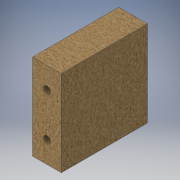
# Autodesk Inventor part: KugelRadStützen
Saved by Autodesk Inventor 2017 SP1 (Build 210196100, 196)
## iProperties
Part Number: KugelRadStützen
Material: Generisch
Document SubType Name: Modeling
Designer: Alex
Density: 1 g/cm^3
Appearance: Vorgabe
Author: Alex
Autodesk Inventor part; units mm, degrees
ref_plane "YZ Plane" through (0, 0, 0) normal (1, 0, 0) x (0, 1, 0)
ref_plane "XZ Plane" through (0, 0, 0) normal (0, 1, 0) x (-1, 0, 0)
ref_plane "XY Plane" through (0, 0, 0) normal (0, 0, 1) x (1, 0, 0)
sketch "Skizze1" plane through (0, 0, 0) normal (0, 1, 0) x (-1, 0, 0)
  line L0 (0, 0) -> (10, 0)
  line L1 (10, 0) -> (10, -30)
  line L2 (10, -30) -> (0, -30)
  line L3 (0, -30) -> (0, 0)
  dimension "d0" = 10
  dimension "d1" = 30
  constraints: 8 end point, 2 parallel, 1 horizontal, 1 perpendicular
  measures "d0" distance of L1.end L2.end
  measures "d1" distance of L0.end L1.end
extrude "Extrusion1" add sketch "Skizze1" along normal blind 30
sketch "Skizze2" plane through (0, 30, 0) normal (0, 1, 0) x (1, 0, 0)
  line L0 (-10, 0) -> (0, 0) projected
  line L1 (0, 0) -> (0, 30) projected
  point P0 (-5, 4.75)
  point P1 (-5, 25.25)
  dimension "d4" = 20.5
  dimension "d5" = 4.75
  dimension "d6" = 5
  constraints: 1 vertical alignment
  measures "d4" distance of point (-5, 25.25) point (-5, 4.75)
  measures "d5" distance from line of L0 point (-5, 4.75)
  measures "d6" distance from line of L1 point (-5, 4.75)
hole "Bohrung1" at (-5, 30, -4.75) at (-5, 30, -25.25) direction (0, -1, 0) diameter 2 depth 10 tip angle 118
sketch "Skizze4" plane through (0, 0, 0) normal (0, -1, 0) x (1, 0, 0)
  line L0 (0, 0) -> (-10, 0) projected
  line L1 (0, -30) -> (0, 0) projected
  point P0 (-5, -22.5)
  point P1 (-5, -7.5)
  dimension "d21" = 15
  dimension "d22" = 7.5
  dimension "d23" = 5
  constraints: 1 vertical alignment
  measures "d21" distance of point (-5, -7.5) point (-5, -22.5)
  measures "d22" distance from line of L0 point (-5, -7.5)
  measures "d23" distance from line of L1 point (-5, -7.5)
hole "Bohrung3" at (-5, 0, -22.5) at (-5, 0, -7.5) direction (0, 1, 0) diameter 2.5 depth 10 tip angle 118
